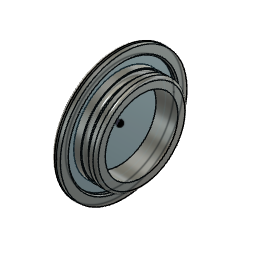
Blanking Plate v2 (Autodesk Fusion 360 design; units mm, degrees)
Autodesk Fusion 360 part; units mm, degrees
sketch "Sketch1" plane through (0, 0, 0) normal (1, 0, 0) x (0, 0, -1)
  circle A0 centre (0, 0) radius 21
  dimension "d1" = 42
  constraint coincident A0.centre origin
  measures "d1" diameter of A0
extrude "Extrude1" add sketch "Sketch1" along normal blind 3.2
sketch "Sketch2" plane through (3.2, 0, 0) normal (1, 0, 0) x (0, 0, -1)
  circle A0 centre (0, 0) radius 21
  circle A1 centre (0, 0) radius 19
  dimension "d4" = 38
  constraint concentric A0 A1
  measures "d4" diameter of A1
extrude "Extrude2" add sketch "Sketch2" along normal blind 3.6 contours A1
sketch "Sketch3" plane through (6.8, 0, 0) normal (1, 0, 0) x (0, 0, -1)
  circle A0 centre (0, 0) radius 19
  circle A1 centre (0, 0) radius 21
  dimension "d7" = 42
  constraint concentric A0 A1
  measures "d7" diameter of A1
extrude "Extrude3" add sketch "Sketch3" along normal blind 3.2 contours A0 | A1
fillet "Fillet1" radius 1.5 2 edges at (3.2, 6.8707, 17.7142) (6.8, -6.8707, 17.7142)
sketch "Sketch4" plane through (0, 0, 0) normal (-1, 0, 0) x (0, 0, 1)
  circle A0 centre (0, 0) radius 21
  circle A1 centre (0, 0) radius 28.9
  dimension "d11" = 57.8
  constraint coincident A0.centre A1.centre
  measures "d11" diameter of A1
extrude "Extrude4" add sketch "Sketch4" along normal blind 2.4 contours A0 | A1
sketch "Sketch5" plane through (0, 0, 0) normal (1, 0, 0) x (0, 0, -1)
  circle A0 centre (0, 0) radius 28.9
  circle A1 centre (0, 0) radius 21
  circle A2 centre (0, 0) radius 24.7
  dimension "d14" = 49.4
  constraint concentric A0 A2
  measures "d14" diameter of A2
extrude "Extrude5" add sketch "Sketch5" along normal blind 1.8 contours A0
sketch "Sketch6" plane through (10, 0, 0) normal (1, 0, 0) x (0, 0, -1)
  circle A0 centre (0, 0) radius 21
  circle A1 centre (0, 0) radius 19
  circle A2 centre (0, 0) radius 16.6
  dimension "d17" = -2.4
extrude "Extrude6" cut sketch "Sketch6" against normal blind 10 contours A2
fillet "Fillet2" radius 1.2 1 edges at (10, -7.5939, 19.5789)
fillet "Fillet3" radius 1.6 1 edges at (-2.4, -10.4507, -26.9443)
fillet "Fillet4" radius 0.6 1 edges at (1.8, 8.9319, 23.0285)
equation "d4 = 41 mm - 3 mm"
